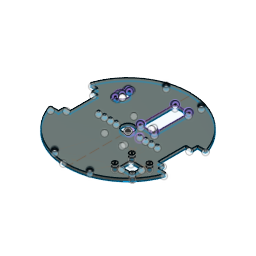
FEKTBOT_upper_ver_1_2 (Autodesk Fusion 360 design; units mm, degrees)
Autodesk Fusion 360 part; units mm, degrees
sketch "podklad" plane through (0, 0, 0) normal (0, 1, 0) x (1, 0, 0)
  line L0 (45, -67.4927) -> (75, -67.4927) construction
  line L1 (-75.0372, -23.4927) -> (-85, -23.4927)
  arc A0 (96.7123, 33.4364) -> (98.5902, 36.1245) centre (96.7123, 35.4364) ccw
  line L2 (45, -38.4927) -> (45, -67.4927) construction
  line L3 (85, -33.4277) -> (85, -23.4927)
  line L4 (-75.0372, -23.4927) -> (-75.0372, 23.5073)
  line L5 (74.9628, -23.4927) -> (74.9628, 23.5073)
  line L6 (0, 105) -> (0, -105) construction
  line L7 (-85, 23.5073) -> (-75.0372, 23.5073)
  arc A1 (-98.5902, 36.1245) -> (-96.7123, 33.4364) centre (-96.7123, 35.4364) ccw
  arc A2 (-96.7154, -33.4277) -> (-98.5934, -36.1156) centre (-96.7154, -35.4277) ccw
  line L8 (74.9628, -23.4927) -> (85, -23.4927)
  line L9 (85, 23.5073) -> (74.9628, 23.5073)
  line L10 (-85, 33.4364) -> (-85, 23.5073)
  arc A3 (-98.5934, -36.1156) -> (98.5934, -36.1156) centre (0, 0) ccw
  line L11 (85, 33.4364) -> (85, 23.5073)
  line L12 (96.7123, 33.4364) -> (85, 33.4364)
  line L13 (-96.7154, -33.4277) -> (-85, -33.4277)
  arc A4 (98.5934, -36.1156) -> (96.7154, -33.4277) centre (96.7154, -35.4277) ccw
  line L14 (75, -67.4927) -> (75, -38.4927) construction
  arc A5 (98.5902, 36.1245) -> (15, 103.923) centre (0, 0) ccw
  arc A6 (15, 103.923) -> (-15, 103.923) centre (0, 0) ccw
  arc A7 (-15, 103.923) -> (-98.5902, 36.1245) centre (0, 0) ccw
  circle A8 centre (75, -38.4927) radius 1.1
  line L15 (75, -38.4927) -> (45, -38.4927) construction
  line L16 (-96.7123, 33.4364) -> (-85, 33.4364)
  circle A9 centre (75, -67.4927) radius 1.1
  circle A10 centre (45, -38.4927) radius 1.1
  line L17 (96.7154, -33.4277) -> (85, -33.4277)
  line L18 (-85, -33.4277) -> (-85, -23.4927)
  circle A11 centre (45, -67.4927) radius 1.1
  line L19 (51, -45) -> (69, -45)
  line L20 (70, -46) -> (70, -62)
  line L21 (69, -63) -> (51, -63)
  line L22 (50, -62) -> (50, -46)
  circle A12 centre (-30, -94.9953) radius 1.85
  circle A13 centre (30, -94.9953) radius 1.85
  circle A14 centre (-29.9934, 95.0047) radius 1.85
  circle A15 centre (29.9934, 95.0047) radius 1.85
  circle A16 centre (0, 0) radius 10
  circle A17 centre (-20, 0.003) radius 1.85
  circle A18 centre (-30, 0.0036) radius 1.85
  circle A19 centre (-40, 0.0023) radius 1.85
  circle A20 centre (-50, 0.0036) radius 1.85
  circle A21 centre (50, 0.0036) radius 1.85
  circle A22 centre (40, 0.0023) radius 1.85
  circle A23 centre (30, 0.0036) radius 1.85
  circle A24 centre (20, 0.003) radius 1.85
  arc A25 (51, -45) -> (50, -46) centre (51, -46) ccw
  arc A26 (70, -46) -> (69, -45) centre (69, -46) ccw
  arc A27 (69, -63) -> (70, -62) centre (69, -62) ccw
  arc A28 (50, -62) -> (51, -63) centre (51, -62) ccw
  line L23 (2.5, 0) -> (20, 0)
  line L24 (6, 15) -> (29, 15)
  line L25 (30, 16) -> (30, 74)
  line L26 (29, 75) -> (6, 75)
  line L27 (5, 74) -> (5, 16)
  arc A29 (6, 75) -> (5, 74) centre (6, 74) ccw
  arc A30 (30, 74) -> (29, 75) centre (29, 74) ccw
  arc A31 (29, 15) -> (30, 16) centre (29, 16) ccw
  arc A32 (5, 16) -> (6, 15) centre (6, 16) ccw
  line L28 (-56.6497, 57.6211) -> (-52.6497, 57.6211)
  line L29 (-52.6497, 33.6211) -> (-56.6497, 33.6211)
  line L30 (-56.6497, 33.6211) -> (-56.6497, 35.202)
  line L31 (-56.6497, 54.798) -> (-56.6497, 57.6211)
  line L32 (-52.6497, 57.6211) -> (-52.6497, 54.798)
  line L33 (-52.6497, 35.202) -> (-52.6497, 33.6211)
  arc A33 (-56.6497, 54.798) -> (-56.6497, 35.202) centre (-54.6497, 45) ccw
  arc A34 (-52.6497, 35.202) -> (-52.6497, 54.798) centre (-54.6497, 45) ccw
  point P0 (-7.5, -102.9967)
  point P1 (-82.0372, 22.8073)
  point P2 (-17.0372, -22.7927)
  point P3 (81.9628, 22.8073)
  point P4 (-0.0372, 0.0073)
  point P5 (-82.0372, -22.7927)
  point P6 (16.9628, 27.0073)
  point P7 (16.9628, 22.8073)
  point P8 (-17.0372, 27.0073)
  point P9 (16.9628, -22.7927)
  point P10 (81.9628, -22.7927)
  point P11 (16.9628, -26.9927)
  dimension "d1" = 210
  dimension "d2" = 2
  dimension "d3" = 2
  dimension "d4" = 2
  dimension "d5" = 2
  dimension "d26" = 30
  dimension "d27" = 29
  dimension "d28" = 2.2
  dimension "d29" = 2.2
  dimension "d30" = 2.2
  dimension "d31" = 2.2
  dimension "d32" = 45
  dimension "d33" = 15
  dimension "d39" = 3.7
  dimension "d40" = 20
  dimension "d41" = 3.7
  dimension "d42" = 3.7
  dimension "d43" = 3.7
  dimension "d44" = 20
  dimension "d45" = 30
  dimension "d46" = 40
  dimension "d47" = 3.7
  dimension "d48" = 50
  dimension "d49" = 1
  dimension "d50" = 1
  dimension "d51" = 1
  dimension "d52" = 1
  dimension "d74" = 1
  dimension "d75" = 20
  dimension "d76" = 4
  dimension "d77" = 24
  dimension "d78" = 2
  constraint horizontal L7
  constraint horizontal L1
  constraint horizontal L9
  constraint horizontal L8
  constraint horizontal L16
  constraint vertical L10
  constraint horizontal L13
  constraint vertical L18
  constraint horizontal L17
  constraint vertical L3
  constraint horizontal L12
  constraint vertical L11
  constraint coincident A3.centre A5.centre
  constraint concentric A3 A5
  constraint tangent A2 A3
  constraint tangent A2 L13
  constraint tangent A1 A5
  constraint tangent A1 L16
  constraint tangent A0 L12
  constraint tangent A0 A5
  constraint tangent A4 L17
  constraint tangent A3 A4
  constraint midpoint L6.end A3
  constraint concentric A5 A7
  constraint coincident L6.start A5
  constraint horizontal L15
  constraint vertical L2
  constraint horizontal L0
  constraint vertical L14
  constraint coincident L2.start L15.end
  constraint coincident L14.end A8.centre
  constraint coincident L0.start L2.end
  constraint coincident L0.end L14.start
  constraint vertical L5
  constraint vertical L4
  constraint coincident L6.start A6
  constraint horizontal L19
  constraint vertical L20
  constraint horizontal L21
  constraint vertical L22
  constraint concentric A3 A16
  constraint symmetric L6 A17 A24
  constraint symmetric L6 A18 A23
  constraint symmetric L6 A19 A22
  constraint symmetric L6 A20 A21
  constraint tangent L19 A25
  constraint tangent L22 A25
  constraint tangent L19 A26
  constraint tangent L20 A26
  constraint tangent L20 A27
  constraint tangent L21 A27
  constraint tangent L21 A28
  constraint tangent L22 A28
  constraint horizontal L24
  constraint vertical L25
  constraint horizontal L26
  constraint vertical L27
  constraint tangent L26 A29
  constraint tangent L27 A29
  constraint tangent L25 A30
  constraint tangent L26 A30
  constraint equal A29 A30
  constraint tangent L24 A31
  constraint tangent L25 A31
  constraint equal A29 A31
  constraint tangent L24 A32
  constraint tangent L27 A32
  constraint equal A29 A32
  constraint horizontal L28
  constraint vertical L32
  constraint horizontal L29
  constraint vertical L30
  constraint collinear L30 L31
  constraint coincident L33.start A33
  constraint collinear L32 L33
  constraint concentric A33 A34
  measures "d1" diameter of A5 L6
  measures "d2" radius of A2
  measures "d3" radius of A1
  measures "d4" radius of A0
  measures "d5" radius of A4
  measures "d26" distance of L2.start L14.end
  measures "d27" distance of L0.end L14.end
  measures "d28" diameter of A10
  measures "d29" diameter of A8
  measures "d30" diameter of A11
  measures "d31" diameter of A9
  measures "d32" distance of L2.start L6
  measures "d33" distance of L2.start L8
  measures "d39" diameter of A13
  measures "d40" diameter of A16
  measures "d41" diameter of A17
  measures "d42" diameter of A18
  measures "d43" diameter of A19
  measures "d44" distance of L6 A17.centre
  measures "d45" distance of L6 A18.centre
  measures "d46" distance of L6 A19.centre
  measures "d47" diameter of A20
  measures "d48" distance of L6 A20.centre
  measures "d49" radius of A25
  measures "d50" radius of A26
  measures "d51" radius of A27
  measures "d52" radius of A28
  measures "d57" diameter of L1.end
  measures "d74" radius of A29
  measures "d75" diameter of A33
  measures "d76" distance of L28.start L28.end
  measures "d77" distance of L28.start L29.end
  measures "d78" distance of A33.centre L32
extrude "Extrude1" add sketch "podklad" along normal blind 5
sketch "diry_hlavy_sroubu" plane through (0, 5, 0) normal (0, 1, 0) x (-1, 0, 0)
  circle A0 centre (29.9934, -95.0047) radius 1.85
  circle A1 centre (-29.9934, -95.0047) radius 1.85
  circle A2 centre (0, 0) radius 10
  circle A3 centre (40, -0.0023) radius 1.85
  circle A4 centre (-30, -0.0036) radius 1.85
  circle A5 centre (30, -0.0036) radius 1.85
  arc A6 (-51, 45) -> (-50, 46) centre (-51, 46) ccw
  line L0 (-51, 45) -> (-69, 45)
  arc A7 (-70, 46) -> (-69, 45) centre (-69, 46) ccw
  line L1 (-70, 46) -> (-70, 62)
  arc A8 (-69, 63) -> (-70, 62) centre (-69, 62) ccw
  line L2 (-69, 63) -> (-51, 63)
  arc A9 (-50, 62) -> (-51, 63) centre (-51, 62) ccw
  line L3 (-50, 62) -> (-50, 46)
  circle A10 centre (-45, 67.4927) radius 1.1
  circle A11 centre (-30, 94.9953) radius 1.85
  circle A12 centre (-50, -0.0036) radius 1.85
  circle A13 centre (-45, 38.4927) radius 1.1
  circle A14 centre (-75, 67.4927) radius 1.1
  circle A15 centre (50, -0.0036) radius 1.85
  circle A16 centre (30, 94.9953) radius 1.85
  circle A17 centre (-40, -0.0023) radius 1.85
  circle A18 centre (-20, -0.003) radius 1.85
  circle A19 centre (20, -0.003) radius 1.85
  circle A20 centre (-75, 38.4927) radius 1.1
  arc A21 (96.7154, 33.4277) -> (98.5934, 36.1156) centre (96.7154, 35.4277) ccw
  arc A22 (98.5934, 36.1156) -> (-98.5934, 36.1156) centre (0, 0) ccw
  arc A23 (-98.5934, 36.1156) -> (-96.7154, 33.4277) centre (-96.7154, 35.4277) ccw
  line L4 (-96.7154, 33.4277) -> (-85, 33.4277)
  line L5 (-85, 33.4277) -> (-85, 23.4927)
  line L6 (-85, 23.4927) -> (-74.9628, 23.4927)
  line L7 (-74.9628, 23.4927) -> (-74.9628, -23.5073)
  line L8 (-74.9628, -23.5073) -> (-85, -23.5073)
  line L9 (-85, -23.5073) -> (-85, -33.4364)
  line L10 (-85, -33.4364) -> (-96.7123, -33.4364)
  arc A24 (-96.7123, -33.4364) -> (-98.5902, -36.1245) centre (-96.7123, -35.4364) ccw
  arc A25 (-98.5902, -36.1245) -> (98.5902, -36.1245) centre (0, 0) ccw
  arc A26 (98.5902, -36.1245) -> (96.7123, -33.4364) centre (96.7123, -35.4364) ccw
  line L11 (96.7123, -33.4364) -> (85, -33.4364)
  line L12 (85, -33.4364) -> (85, -23.5073)
  line L13 (85, -23.5073) -> (75.0372, -23.5073)
  line L14 (75.0372, -23.5073) -> (75.0372, 23.4927)
  line L15 (75.0372, 23.4927) -> (85, 23.4927)
  line L16 (85, 23.4927) -> (85, 33.4277)
  line L17 (85, 33.4277) -> (96.7154, 33.4277)
  circle A27 centre (29.9934, -95.0047) radius 3.5
  circle A28 centre (-29.9934, -95.0047) radius 3.5
  circle A29 centre (30, 94.9953) radius 3.5
  circle A30 centre (-30, 94.9953) radius 3.5
  line L18 (-5, -16) -> (-5, -74)
  line L19 (-6, -75) -> (-29, -75)
  line L20 (-30, -74) -> (-30, -16)
  line L21 (-29, -15) -> (-6, -15)
  arc A31 (-5, -16) -> (-6, -15) centre (-6, -16) ccw
  arc A32 (-6, -75) -> (-5, -74) centre (-6, -74) ccw
  arc A33 (-30, -74) -> (-29, -75) centre (-29, -74) ccw
  arc A34 (-29, -15) -> (-30, -16) centre (-29, -16) ccw
  line L22 (52.6497, -35.202) -> (52.6497, -33.6211)
  line L23 (52.6497, -33.6211) -> (56.6497, -33.6211)
  line L24 (56.6497, -33.6211) -> (56.6497, -35.202)
  arc A35 (56.6497, -54.798) -> (56.6497, -35.202) centre (54.6497, -45) ccw
  line L25 (56.6497, -54.798) -> (56.6497, -57.6211)
  line L26 (56.6497, -57.6211) -> (52.6497, -57.6211)
  line L27 (52.6497, -57.6211) -> (52.6497, -54.798)
  arc A36 (52.6497, -35.202) -> (52.6497, -54.798) centre (54.6497, -45) ccw
  dimension "d55" = 7
  dimension "d56" = 7
  dimension "d57" = 7
  dimension "d58" = 7
  constraint concentric A0 A27
  constraint concentric A1 A28
  constraint concentric A16 A29
  constraint concentric A11 A30
  measures "d55" diameter of A27
  measures "d56" diameter of A28
  measures "d57" diameter of A29
  measures "d58" diameter of A30
extrude "Extrude3" cut sketch "diry_hlavy_sroubu" against normal blind 3 contours A27 | A28 | A29 | A30
sketch "sloupky_displej" plane through (0, 5, 0) normal (0, 1, 0) x (-1, 0, 0)
  circle A0 centre (-45, 38.4927) radius 4
  circle A1 centre (-75, 38.4927) radius 4
  circle A2 centre (-45, 67.4927) radius 4
  circle A3 centre (-75, 67.4927) radius 4
  circle A4 centre (-45, 67.4927) radius 1.1
  circle A5 centre (-75, 67.4927) radius 1.1
  circle A6 centre (-75, 38.4927) radius 1.1
  circle A7 centre (-45, 38.4927) radius 1.1
  point P0 (-45, 38.4927)
  point P1 (-75, 38.4927)
  point P2 (-45, 67.4927)
  point P3 (-75, 67.4927)
  point P4 (-43.9, 67.4927)
  point P5 (-73.9, 67.4927)
  point P6 (-73.9, 38.4927)
  point P7 (-43.9, 38.4927)
  dimension "d63" = 8
  dimension "d64" = 8
  dimension "d65" = 8
  dimension "d66" = 8
  constraint coincident P0 A0.centre
  constraint coincident P1 A1.centre
  constraint coincident P2 A2.centre
  constraint coincident P3 A3.centre
  constraint coincident A4 P4
  constraint concentric A3 A5
  constraint coincident A5 P5
  constraint coincident A6 P6
  constraint coincident A7 P7
  measures "d63" diameter of A0
  measures "d64" diameter of A1
  measures "d65" diameter of A2
  measures "d66" diameter of A3
extrude "Extrude4" add sketch "sloupky_displej" along normal blind 5
